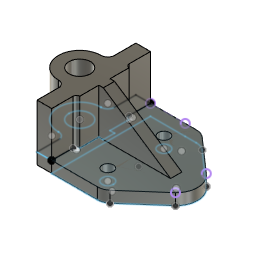
A3 object var finala v2 (Autodesk Fusion 360 design; units mm, degrees)
Autodesk Fusion 360 part; units mm, degrees
sketch "Sketch1" plane through (0, 0, 0) normal (0, 0, 1) x (1, 0, 0)
  line L0 (7.2632, 44) -> (-2.5, 44)
  line L1 (-33.5, 44) -> (-33.5, -44)
  line L2 (-2.5, -44) -> (7.2632, -44)
  circle A0 centre (-2.5, 25) radius 5
  circle A1 centre (-2.5, -25) radius 5
  spline S0 degree 5 poles (15.5225, 41.0391) (16.7241, 39.9848) (19.1273, 37.876) (22.7321, 34.7129) (27.5386, 30.4953) (33.5466, 25.2234) (38.3531, 21.0059) (41.9579, 17.8428) (44.3611, 15.734) (45.5627, 14.6796) knots 0 0 0 0 0 0 0.2 0.4 0.6 0.8 1 1 1 1 1 1
  spline S1 degree 5 poles (15.5202, -41.041) (16.7627, -39.9506) (19.2475, -37.7697) (22.9748, -34.4984) (27.9445, -30.1366) (34.1566, -24.6845) (39.1263, -20.3227) (42.8536, -17.0514) (45.3384, -14.8705) (46.5808, -13.7801) knots 0 0 0 0 0 0 0.2 0.4 0.6 0.8 1 1 1 1 1 1
  line L3 (-33.5, 44) -> (-2.5, 44)
  arc A2 (15.5225, 41.0391) -> (7.2632, 44) centre (7.2632, 31) ccw
  line L4 (-33.5, -44) -> (-2.5, -44)
  arc A3 (7.2632, -44) -> (15.5202, -41.041) centre (7.2632, -31) ccw
  arc A4 (45.4664, -14.7583) -> (45.5626, 14.6797) centre (33.5, 0) ccw
  dimension "d2" = 88
  dimension "d6" = 10
  dimension "d10" = 19
  dimension "d15" = 10
  dimension "d17" = 13
  constraint horizontal L0
  constraint perpendicular L0 L1
  constraint parallel L0 L2
  constraint coincident S0.end A4
  constraint coincident S1.end A4
  constraint coincident S0 A4.end
  constraint coincident S1 A4.start
  measures "d2" distance of L1.start L1.end
  measures "d6" diameter of A0
  measures "d10" radius of A4
  measures "d15" diameter of A1
  measures "d17" radius of A3
extrude "Extrude1" add sketch "Sketch1" along normal blind 10 contours L0 L1 L2 S0 S1 L3 A2 L4 A3 A4 makes body 1
sketch "Sketch2" plane through (0, 0, 10) normal (0, 0, 1) x (-1, 0, 0)
  circle A0 centre (2.5, -25) radius 5
  circle A1 centre (2.5, 25) radius 5
  arc A2 (-15.5225, -41.0391) -> (-7.2632, -44) centre (-7.2632, -31) ccw
  line L0 (-7.2632, -44) -> (33.5, -44)
  line L1 (33.5, -44) -> (33.5, 44)
  line L2 (33.5, 44) -> (-7.2632, 44)
  arc A3 (-7.2632, 44) -> (-15.5202, 41.041) centre (-7.2632, 31) ccw
  line L3 (-15.5202, 41.041) -> (-46.5808, 13.7801)
  arc A4 (-46.5808, 13.7801) -> (-45.5626, -14.6797) centre (-33.5, 0) ccw
  line L4 (-45.5626, -14.6797) -> (-15.5225, -41.0391)
  line L5 (33.5, -44) -> (46.5, -44)
  line L6 (46.5, 44) -> (33.5, 44)
  line L7 (33.5, -44) -> (2.5, -44) construction
  line L8 (26.5, -4.9934) -> (30.5, -4.9934)
  line L9 (30.5, -4.9934) -> (30.5, -22.003)
  line L10 (26.5, 5.0066) -> (30.5, 5.0066)
  line L11 (30.5, 5.0066) -> (30.5, 22)
  arc A5 (30.5, 22) -> (33.5, 25.0017) centre (30.5, 25) ccw
  arc A6 (33.5, -25) -> (30.5, -22) centre (30.5, -25) ccw
  line L12 (33.5, -44) -> (33.5, -25)
  line L13 (33.5, 25) -> (33.5, 44)
  line L14 (26.5, -4.9934) -> (26.5, 5.0066)
  circle A7 centre (52.5, 0) radius 9.5
  arc A8 (46.5, 23.7362) -> (52.5, 19.0134) centre (52.3628, 25.0118) ccw
  arc A9 (52.589, -18.9998) -> (46.5, -24.9991) centre (52.5, -24.9991) ccw
  arc A10 (52.411, -18.9998) -> (52.5, 19) centre (52.5, 0) ccw
  line L15 (52.5, 19.0134) -> (52.5, 19)
  line L16 (52.5, -18.9991) -> (52.5, -19)
  line L17 (46.5, -44) -> (46.5, -24.9991)
  line L18 (46.5, 23.7362) -> (46.5, 44)
  dimension "d18" = 13
  dimension "d35" = 10
  dimension "d36" = 3
  dimension "d37" = 3
  dimension "d40" = 19
  dimension "d41" = 19
  dimension "d42" = 6
  dimension "d43" = 6
  dimension "d48" = 4
  constraint coincident L0.end L1.start
  constraint perpendicular L1 L5
  constraint perpendicular L5 L17
  constraint coincident L1.end L2.start
  constraint tangent A6 L12
  constraint coincident L1 A5.end
  constraint coincident L9 A6.end
  constraint coincident L1 A6.start
  constraint collinear L12 L13
  constraint coincident A5 L13.start
  constraint concentric A7 A10
  constraint coincident A9.start A10
  constraint coincident A9 A10.start
  constraint coincident A8.start L17
  constraint collinear L15 L16
  constraint coincident A7.centre L15
  constraint coincident A9 L16.start
  constraint coincident A10 L16.end
  constraint collinear L17 L18
  measures "d18" distance of L0.end L5.end
  measures "d35" distance of L8 L10
  measures "d36" radius of A5
  measures "d37" radius of A6
  measures "d40" radius of A10
  measures "d41" diameter of A7
  measures "d42" radius of A8
  measures "d43" radius of A9
  measures "d48" distance of L11 L14
extrude "Extrude2" add sketch "Sketch2" against normal blind 10 separate body contours L1 L5 L6 L12 L13 A8 A9 A10 L15 L17 L18 makes body 2
extrude "Extrude3" add sketch "Sketch2" along normal blind 40 contours L1 L5 L6 A5 L12 L13 A8 A9 A10 L15 L17 L18 | L1 L8 L9 L10 L11 A5 A6 L14 bodies 2 1
draft "Draft1" angle 56.3 neutral plane through (0, 0, 50) pull (0, 0, 1) 1 faces at (-26.5, 1.6601, 23.3333) on bodies 2
named bodies: "A3 final object"
